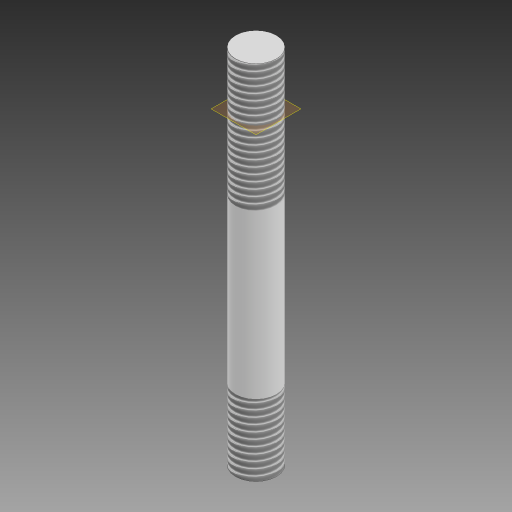
# Autodesk Inventor part: HUDSON-1-49A
Saved by Autodesk Inventor 2024.2 (Build 282272000, 272)
## iProperties
Created: 2024-10-10
Part Number: HUDSON-1-49A
Material: Generic
Document SubType Name: Modeling
Designer: Precisión-05
Density: 1 g/cm^3
Appearance: Default
Author: Precisión-05
Autodesk Inventor part; units mm, degrees
ref_plane "YZ Plane" through (0, 0, 0) normal (1, 0, 0) x (0, 1, 0)
ref_plane "XZ Plane" through (0, 0, 0) normal (0, 1, 0) x (-1, 0, 0)
sketch "Sketch1" plane through (0, 0, 0) normal (1, 0, 0) x (0, 1, 0)
  line L0 (-4, -35.5) -> (4, -35.5)
  line L1 (4, -35.5) -> (4, 35.5)
  line L2 (4, 35.5) -> (-4, 35.5)
  line L3 (-4, 35.5) -> (-4, -35.5)
  line L4 (-4, -35.5) -> (4, 35.5) construction
  line L5 (4, -35.5) -> (-4, 35.5) construction
  line L6 (0, 35.5) -> (0, -35.5)
  point P0 (0, 0)
  dimension "d0" = 8
  dimension "d1" = 71
  constraints: 14 end point, 4 midpoint, 2 parallel, 1 horizontal, 1 perpendicular
  measures "d0" distance of L2.end L1.end
  measures "d1" distance of L1.end L0.end
revolve "Revolution1" add sketch "Sketch1" angle 360 about axis through (0, 0, 35.5) along (0, 0, -1) contours L6 L2 L1 L0
thread "Thread1" size "M8x1.25" class "6g" standard "ANSI Metric M Profile" length 25
ref_plane "Work Plane1" through (0, 0, 25) normal (0, 0, 1) x (1, 0, 0)
sketch "Sketch3" plane through (0, 0, 25) normal (0, 0, 1) x (1, 0, 0)
  point P0 (0, 0)
thread "Thread2" size "M8x1.25" class "6g" standard "ANSI Metric M Profile" length 14
body "Solid1"
